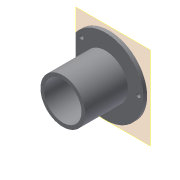
# Autodesk Inventor part: 10_Zeiss_Axiotech_Eypiecemount_Adapter
Saved by Autodesk Inventor 2019 (Build 230136000, 136)
## iProperties
Created: 2019-06-02
Part Number: 10_Zeiss_Axiotech_Eypiecemount_Adapter
Material: Generic
Document SubType Name: Modeling
Designer: diederichbenedict
Density: 1 g/cm^3
Appearance: Default
Author: diederichbenedict
Autodesk Inventor part; units mm, degrees
ref_plane "YZ Plane" through (0, 0, 0) normal (1, 0, 0) x (0, 1, 0)
ref_plane "XZ Plane" through (0, 0, 0) normal (0, 1, 0) x (-1, 0, 0)
ref_plane "XY Plane" through (0, 0, 0) normal (0, 0, 1) x (1, 0, 0)
ref_plane "Work Plane1" through (0, 0, 0) normal (0, 0, 1) x (1, 0, 0)
sketch "Sketch1" plane through (0, 0, 0) normal (0, 0, 1) x (1, 0, 0)
  circle A0 centre (27.1062, 0) radius 1.75 construction
  circle A1 centre (-19.5414, -18) radius 1.75 construction
  circle A2 centre (-19.5414, 18) radius 1.75 construction
  arc A3 (-24.1905, -18.9934) -> (-24.1905, 18.9934) centre (0.3095, 0) ccw projected
  circle A4 centre (0.3095, 0) radius 15.25 projected
  circle A5 centre (-19.5414, 18) radius 1.75 projected
  circle A6 centre (-19.5414, -18) radius 1.75 projected
  circle A7 centre (27.1062, 0) radius 1.75 projected
  line L0 (-24.1905, 18.9934) -> (-24.1905, -18.9934) projected
  arc A8 (-24.1905, -18.9934) -> (-24.1905, 18.9934) centre (0.3095, 0) ccw projected
  circle A9 centre (0.3095, 0) radius 15.25
  point P0 (0, 0)
  constraints: 1 centre point, 1 coincident, 1 concentric
extrude "Extrusion1" add sketch "Sketch1" along normal blind 3
sketch "Sketch2" plane through (0, 0, 3) normal (0, 0, 1) x (1, 0, 0)
  circle A0 centre (0.3095, 0) radius 15.25 projected
  circle A1 centre (0.3095, 0) radius 15.3
  circle A2 centre (0.3095, 0) radius 18.3
  point P0 (0, 0)
  dimension "d2" = 30.6
  dimension "d3" = 3
  constraints: 2 centre point, 1 coincident
  measures "d2" diameter of A1
  measures "d3" radial gap between concentric circles of A1 A2
extrude "Extrusion2" add sketch "Sketch2" along normal blind 35 contours A2
body "Solid1"
